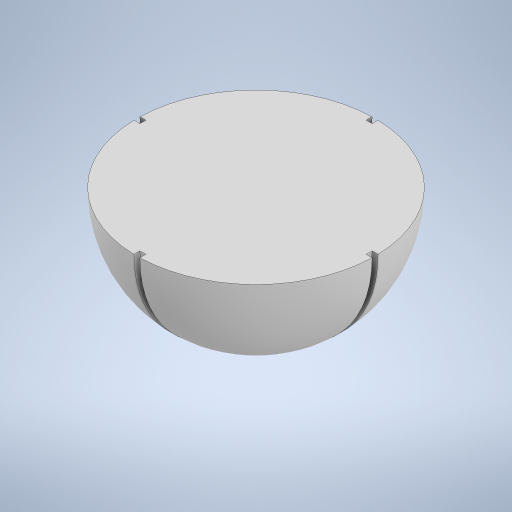
# Autodesk Inventor part: 屋2 base
Saved by Autodesk Inventor 2024 (Build 280153000, 153)
## iProperties
Created: 2024-05-22
Part Number: 屋2 base
Material: 一般
Document SubType Name: Modeling
Designer: User
Density: 1 g/cm^3
Appearance: 預設
Author: User
Autodesk Inventor part; units mm, degrees
ref_plane "YZ Plane" through (0, 0, 0) normal (1, 0, 0) x (0, 1, 0)
ref_plane "XZ Plane" through (0, 0, 0) normal (0, 1, 0) x (-1, 0, 0)
ref_plane "XY Plane" through (0, 0, 0) normal (0, 0, 1) x (1, 0, 0)
sketch "草圖1" plane through (0, 0, 0) normal (0, 1, 0) x (-1, 0, 0)
  circle A0 centre (0, 0) radius 20
  line L0 (0, 20) -> (0, -20)
  dimension "d0" = 40
  constraints: 2 end point, 2 point on circle, 1 centre point, 1 coincident, 1 vertical
  measures "d0" diameter of A0
revolve "迴轉1" add sketch "草圖1" angle 180 about axis through (0, 0, 20) along (0, 0, -1) picked at (-3.0982, -5.903) contours L0 A0
sketch "草圖2" plane through (0, 0, 0) normal (0, 0, 1) x (1, 0, 0)
  line L0 (20, 0) -> (-20, 0) projected
  arc A0 (-20, 0) -> (20, 0) centre (0, 0) ccw
  arc A1 (-20, 0) -> (20, 0) centre (0, 0) ccw projected
  arc A2 (-19, 0) -> (19, 0) centre (0, 0) ccw
  line L1 (-19, 0) -> (-20, 0)
  line L2 (19, 0) -> (20, 0)
  dimension "d2" = 1
  constraints: 4 end point, 4 point on circle, 2 centre point, 2 concentric, 2 point on line, 1 collinear, 1 horizontal
  measures "d2" radial gap between concentric circles of A0 A2
extrude "擠出1" cut sketch "草圖2" along normal mid plane 1 contours A0 L0 A2
sketch "草圖3" plane through (0, 0, 0) normal (1, 0, 0) x (0, 1, 0)
  line L0 (0, 0.5) -> (0, 20) projected
  line L1 (0, -20) -> (0, -0.5) projected
  arc A0 (0, 19) -> (0, -19) centre (0, 0) ccw
  arc A1 (0, 20) -> (0, -20) centre (0, 0) ccw
  line L2 (0, 20) -> (0, 19)
  line L3 (0, -20) -> (0, -19)
  dimension "d5" = 1
  constraints: 4 end point, 4 point on circle, 2 centre point, 2 point on line, 1 collinear, 1 concentric, 1 vertical
  measures "d5" radial gap between concentric circles of A1 A0
extrude "擠出2" cut sketch "草圖3" along normal mid plane 1
